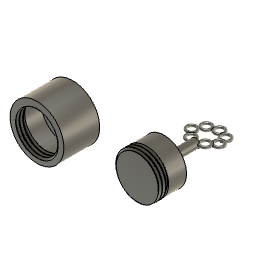
Flower Vase_ v1 (Autodesk Fusion 360 design; units mm, degrees)
Autodesk Fusion 360 part; units mm, degrees
cylinder "CylinderPrimitive2" add diameter 60 height 40 placed x (1, 0, 0) y (0, 0, -1) z (0, 1, 0) at (0, 0, 0) makes body 1
cylinder "CylinderPrimitive3" add diameter 50 height 30 placed x (1, 0, 0) y (0, 0, -1) z (0, 1, 0) at (0, 0, 0) separate body makes body 2
thread "Thread1" "ISO Metric profile 50.0 M50x4 6g" major diameter 49.7025 minor diameter 45.1258 pitch 4 angle 60 modelled right hand crest width 0.569 on face at (24.8758, 10, 2.4892) from (0, 0, 0) to (0, 10, 0) crest through (24.8513, -1, 0) on bodies 2
copy_body "CopyPasteBodies1" bodies 1 makes body 3
copy_body "CopyPasteBodies2" bodies 2 makes body 4
move_body "Move1" bodies 4 to x (1, 0, 0) y (0, 1, 0) z (0, 0, 1) at (98.46, 13.7805, -0.3722)
combine "Combine1" operation cut target body 3 tool bodies 2
cylinder "CylinderPrimitive4" add diameter 10 height 35 placed x (1, 0, 0) y (0, 0, -1) z (0, 1, 0) at (98.46, 43.7805, -0.3722) bodies 4
torus "TorusPrimitive1" add centre line diameter 10 section diameter 3 placed x (1, 0, 0) y (0, 1, 0) z (0, 0, 1) at (94, 78, 0) separate body makes body 5
move_body "MoveFace1" bodies 5 to x (1, 0, 0) y (0, 1, 0) z (0, 0, 1) at (-3.4542, 3.5671, -0.4149) on bodies 5
sketch "Sketch6" plane through (0, 0, 0) normal (1, 0, 0) x (0, 1, 0)
sketch "Sketch7" plane through (0, 0, 0) normal (1, 0, 0) x (0, 1, 0)
torus "TorusPrimitive2" add centre line diameter 10 section diameter 3 placed x (1, 0, 0) y (0, 1, 0) z (0, 0, 1) at (92, 87, 0) separate body makes body 6
move_body "MoveFace2" bodies 6 to x (1, 0, 0) y (0, 1, 0) z (0, 0, 1) at (-8.8654, 2.747, 0) on bodies 6
copy_body "CopyPasteBodies3" bodies 6 makes body 7
move_body "Move2" bodies 7 to x (1, 0, 0) y (0, 1, 0) z (0, 0, 1) at (5.0132, 11.4744, -1.0319)
copy_body "CopyPasteBodies4" bodies 7 makes body 8
move_body "Move3" bodies 8 to x (1, 0, 0) y (0, 1, 0) z (0, 0, 1) at (10.931, 3.6975, -0.2866)
copy_body "CopyPasteBodies5" bodies 8 makes body 9
move_body "Move4" bodies 9 to x (1, 0, 0) y (0, 1, 0) z (0, 0, 1) at (10.844, -4.027, 0.4242)
copy_body "CopyPasteBodies6" bodies 9 makes body 10
move_body "Move5" bodies 10 to x (1, 0, 0) y (0, 1, 0) z (0, 0, 1) at (2.9335, -10.4268, 0.9746)
copy_body "CopyPasteBodies7" bodies 10 makes body 11
move_body "Move6" bodies 11 to x (1, 0, 0) y (0, 1, 0) z (0, 0, 1) at (-6.8068, -8.333, 0.7338)
combine "Combine2" operation add target body 4 tool bodies 5 6 7 8 9 10 11
hidden bodies 1
equation "cylinder_diameter = 60 mm"
equation "cylinder_height = 40 mm"
equation "d7 = cylinder_height"
equation "d8 = cylinder_diameter"
equation "d10 = cylinder_height - 10 mm"
equation "d11 = cylinder_diameter - 10 mm"
